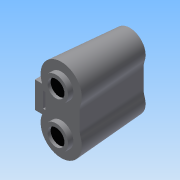
# Autodesk Inventor part: head1
Saved by Autodesk Inventor 2015 (Build 190159000, 159)
## iProperties
Created: 2015-06-18
Part Number: head1
Material: Générique
Document SubType Name: Modeling
Designer: Gregwar
Density: 1 g/cm^3
Appearance: Par défaut
Author: Gregwar
Autodesk Inventor part; units mm, degrees
ref_plane "YZ Plane" through (0, 0, 0) normal (1, 0, 0) x (0, 1, 0)
ref_plane "XZ Plane" through (0, 0, 0) normal (0, 1, 0) x (-1, 0, 0)
ref_plane "XY Plane" through (0, 0, 0) normal (0, 0, 1) x (1, 0, 0)
sketch "Esquisse7" plane through (0, 0, 0) normal (0, 1, 0) x (-1, 0, 0)
  circle A0 centre (0, 0) radius 15
  circle A1 centre (0, -39.9666) radius 15
  line L0 (13, -7.4833) -> (-13, -7.4833)
  line L1 (-13, -7.4833) -> (-13, -32.4833)
  line L2 (-13, -32.4833) -> (13, -32.4833)
  line L3 (13, -32.4833) -> (13, -7.4833)
  dimension "d39" = 30
  dimension "d40" = 25
  dimension "d41" = 26
  constraints: 8 end point, 4 point on circle, 2 centre point, 2 parallel, 1 coincident, 1 equal radius, 1 horizontal, 1 perpendicular
  measures "d39" diameter of A0
  measures "d40" distance of L0.end L1.end
  measures "d41" distance of L1.end L2.end
extrude "Extrusion7" add sketch "Esquisse7" along normal blind 65
sketch "Esquisse8" plane through (-13, 0, -32.4833) normal (-1, 0, 0) x (0, 0, 1)
  line L0 (0, 0) -> (25, 0) construction
  line L1 (25, 0) -> (25, 65) construction
  line L2 (0, 65) -> (25, 65) construction
  line L3 (0, 0) -> (0, 65) construction
  line L4 (25, 0) -> (0, 0)
  line L5 (0, 0) -> (0, 65)
  line L6 (0, 65) -> (25, 65)
  line L7 (25, 65) -> (25, 0)
  point P0 (32.4833, 0)
  constraints: 8 end point, 2 parallel, 1 horizontal, 1 perpendicular
extrude "Extrusion8" add sketch "Esquisse8" along normal blind 12
sketch "Esquisse9" plane through (0, 0, 0) normal (0, -1, 0) x (1, 0, 0)
  arc A0 (-13, -32.4833) -> (13, -32.4833) centre (0, -39.9666) ccw construction
  line L0 (13, -7.4833) -> (13, -32.4833) construction
  arc A1 (13, -7.4833) -> (-13, -7.4833) centre (0, 0) ccw construction
  line L1 (-13, -7.4833) -> (-25, -7.4833) construction
  line L2 (-25, -32.4833) -> (-25, -7.4833) construction
  line L3 (-13, -32.4833) -> (-25, -32.4833) construction
  line L4 (-13, -7.4833) -> (-25, -7.4833) construction
  line L5 (-15, -7.4833) -> (-15, -32.4833) construction
  line L6 (-13, -32.4833) -> (-25, -32.4833) construction
  line L7 (-15, -12.7966) -> (-17.3067, -12.7966)
  line L8 (-17.3067, -12.7966) -> (-17.3067, -27.5847)
  line L9 (-17.3067, -27.5847) -> (-15, -27.5847)
  line L10 (-15, -27.5847) -> (-15, -12.7966)
  point P0 (-15, -29.9833)
  dimension "d47" = 10
  constraints: 10 end point, 4 point on line, 2 parallel, 1 horizontal, 1 perpendicular, 1 vertical
  measures "d47" distance between parallel lines of L2 L5
extrude "Extrusion9" cut sketch "Esquisse9" against normal blind 3
sketch "Esquisse10" plane through (0, 0, 0) normal (0, -1, 0) x (1, 0, 0)
  arc A0 (-13, -32.4833) -> (13, -32.4833) centre (0, -39.9666) ccw construction
  line L0 (13, -7.4833) -> (13, -32.4833) construction
  arc A1 (13, -7.4833) -> (-13, -7.4833) centre (0, 0) ccw construction
  line L1 (-13, -7.4833) -> (-25, -7.4833) construction
  line L2 (-25, -32.4833) -> (-25, -7.4833) construction
  line L3 (-13, -32.4833) -> (-25, -32.4833) construction
  circle A2 centre (0, 0) radius 11.5
  circle A3 centre (0, -39.9666) radius 11.5
  arc A4 (-13, -32.4833) -> (13, -32.4833) centre (0, -39.9666) ccw projected
  dimension "d58" = 23
  constraints: 2 centre point, 2 coincident, 1 concentric, 1 equal radius
  measures "d58" diameter of A3
extrude "Extrusion10" add sketch "Esquisse10" along normal blind 5
sketch "Esquisse11" plane through (0, -5, 0) normal (0, -1, 0) x (1, 0, 0)
  circle A0 centre (0, -39.9666) radius 11.5 construction
  circle A1 centre (0, 0) radius 11.5 construction
  circle A2 centre (0, 0) radius 8
  circle A3 centre (0, -39.9666) radius 8
  dimension "d54" = 16
  constraints: 2 centre point, 2 coincident, 1 equal radius
  measures "d54" diameter of A3
extrude "Extrusion11" cut sketch "Esquisse11" against normal blind 3
fillet "Congé6" radius 20 2 edges at (13, 32.5, -7.4833) (13, 32.5, -32.4833)
draft "Dépouille de face1" angle 4 pull direction (0, 1, 0) faces at (13, 21.6667, -17.2095) (13.057, 21.6667, -29.813) (13.2275, 21.6667, -8.6539) (-14.4854, 43.3333, -43.862) (-14.0102, 43.3333, -5.3586) fixed edges at (13, 65, -19.9833) (13.2878, 65, -31.6853) (13.2878, 65, -8.2813) (-1.3678, 65, -54.9041) (-1.3678, 65, 14.9375)
